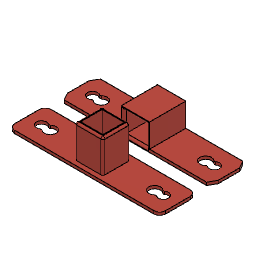
Solenoid v3 (Autodesk Fusion 360 design; units mm, degrees)
Autodesk Fusion 360 part; units mm, degrees
sketch "Sketch1" plane through (0, 0, 0) normal (0, 1, 0) x (1, 0, 0) in component "Solenoid base"
  line L0 (-25.5016, -20.45) -> (57.0484, -20.45)
  line L1 (57.0484, -20.45) -> (57.0484, -0.6062)
  line L2 (57.0484, -0.6062) -> (-25.5016, -0.6062)
  line L3 (-25.5016, -0.6062) -> (-25.5016, -20.45)
  dimension "d1_1_1" = 82.55
  dimension "d2_1_1" = 19.8438
  constraint horizontal L0
  constraint vertical L1
  constraint horizontal L2
  constraint vertical L3
  measures "d1_1_1" distance of L0.start L0.end
  measures "d2_1_1" distance of L0.end L1.end
extrude "Extrude1" add sketch "Sketch1" against normal blind 1.5875 makes body 1 in component "Solenoid base"
sketch "Sketch5" plane through (0, -1.5875, 0) normal (0, -1, 0) x (1, 0, 0) in component "Solenoid base"
  line L0 (15.7734, -11.3) -> (15.7734, 20.45) construction
  line L1 (46.9483, 10.5281) -> (-16.5517, 10.5281) construction
  line L2 (44.3484, 10.5281) -> (49.1109, 10.5281) construction
  arc A0 (47.5032, 8.2625) -> (46.5048, 8.1977) centre (47.0438, 7.6151) ccw
  arc A1 (46.5048, 12.8585) -> (47.5032, 12.7938) centre (47.0438, 13.4411) ccw
  arc A2 (47.5032, 8.2625) -> (47.5032, 12.7938) centre (49.1109, 10.5281) ccw
  arc A3 (46.5048, 12.8585) -> (46.5048, 8.1977) centre (44.3484, 10.5281) ccw
  arc A4 (-14.958, 8.1977) -> (-14.958, 12.8585) centre (-12.8016, 10.5281) ccw
  arc A5 (-15.9564, 12.7938) -> (-15.9564, 8.2625) centre (-17.5641, 10.5281) ccw
  arc A6 (-15.9564, 12.7938) -> (-14.958, 12.8585) centre (-15.497, 13.4411) ccw
  arc A7 (-14.958, 8.1977) -> (-15.9564, 8.2625) centre (-15.497, 7.6151) ccw
  line L3 (49.1109, 10.5281) -> (-12.8016, 10.5281) construction
  line L4 (57.0484, 10.5281) -> (-25.5016, 10.5281) construction
  line L5 (57.0484, 20.45) -> (-25.5016, 20.45)
  line L6 (-25.5016, 20.45) -> (-25.5016, 0.6062)
  line L7 (-25.5016, 0.6062) -> (57.0484, 0.6062)
  line L8 (57.0484, 0.6062) -> (57.0484, 20.45)
  dimension "d33_1_1" = 5.5563
  dimension "d35_1_1" = 1.5875
  dimension "d38_1_1" = 4.7625
  dimension "d40_1_1" = 3.175
  dimension "d2" = 28.575
  constraint coincident L2.end A2.centre
  constraint tangent A0 A2
  constraint horizontal L2
  constraint symmetric L2 A0.end A1.start
  constraint symmetric L2 A0.start A1.end
  constraint symmetric L2 A0 A1
  constraint tangent A0 A3
  constraint coincident L2.start A3.centre
  constraint symmetric L0 A0.end A4.start
  constraint symmetric L0 A0.start A5.end
  constraint symmetric L0 A0 A7
  constraint symmetric L0 A1.end A5.start
  constraint symmetric L0 A1.start A4.end
  constraint symmetric L0 A1 A6
  constraint symmetric L0 A2 A5
  constraint symmetric L0 A3 A4
  constraint coincident A4.centre L3.end
  constraint perpendicular L0 L3
  constraint collinear L1 L3
  constraint collinear L1 L4
  measures "d33_1_1" diameter of A2
  measures "d35_1_1" diameter of A0
  measures "d38_1_1" distance of L2.start L2.end
  measures "d40_1_1" radius of A3
  measures "d2" distance of L0 L2.start
extrude "Extrude12" cut sketch "Sketch5" against normal up to surface (1.5875 mm away) contours A0 A1 A2 A3 | A4 A5 A6 A7 bodies 1 in component "Solenoid base"
sketch "Sketch17" plane through (0, 0, 20.45) normal (0, 0, 1) x (1, 0, 0) in component "Solenoid base"
  line L0 (57.0484, 0) -> (-25.5016, 0)
  line L1 (-25.5016, -1.5875) -> (57.0484, -1.5875)
  line L2 (15.7734, 0) -> (15.7734, 14.8694) construction
  line L3 (15.7734, 0) -> (21.9329, 0)
  line L4 (21.9329, 0) -> (21.9329, 11.303)
  line L5 (21.9329, 11.303) -> (15.7734, 11.303)
  line L6 (9.6139, 0) -> (9.6139, 11.303)
  line L7 (9.6139, 11.303) -> (15.7734, 11.303)
  line L8 (8.0264, 0) -> (8.0264, 12.8905)
  line L9 (8.0264, 12.8905) -> (15.7734, 12.8905)
  line L10 (23.5204, 12.8905) -> (15.7734, 12.8905)
  line L11 (23.5204, -1.5875) -> (23.5204, 12.8905)
  line L12 (15.7734, -1.5875) -> (23.5204, -1.5875)
  line L13 (-25.5016, 0) -> (-25.5016, -1.5875)
  line L14 (57.0484, -1.5875) -> (57.0484, 0)
  dimension "d5" = 11.303
  dimension "d6" = 6.1595
  dimension "d7" = 1.5875
  constraint midpoint L0 L2.start
  constraint perpendicular L0 L2
  constraint horizontal L3
  constraint vertical L4
  constraint horizontal L5
  constraint symmetric L2 L3.end L6.start
  constraint symmetric L2 L4.end L6.end
  constraint symmetric L2 L5.end L7.end
  measures "d5" distance of L3 L5
  measures "d6" distance of L2 L4
extrude "Extrude13" add sketch "Sketch17" against normal up to surface (19.8438 mm away) contours L0 L4 L5 L6 L7 L8 L9 L10 L11 bodies 1 in component "Solenoid base"
sketch "Sketch1 (2)" plane through (0, 0, 0) normal (0, 1, 0) x (1, 0, 0) in component "Solenoid base vertical"
  line L0 (-25.5016, -20.45) -> (57.0484, -20.45)
  line L1 (57.0484, -20.45) -> (57.0484, -0.6062)
  line L2 (57.0484, -0.6062) -> (-25.5016, -0.6062)
  line L3 (-25.5016, -0.6062) -> (-25.5016, -20.45)
  dimension "d1_1_1_1" = 82.55
  dimension "d2_1_1_1" = 19.8438
  constraint horizontal L0
  constraint vertical L1
  constraint horizontal L2
  constraint vertical L3
  measures "d1_1_1_1" distance of L0.start L0.end
  measures "d2_1_1_1" distance of L0.end L1.end
extrude "Extrude1'" add sketch "Sketch1 (2)" against normal blind 1.5875 separate body makes body 2 in component "Solenoid base vertical"
sketch "Sketch5 (2)" plane through (0, -1.5875, 0) normal (0, -1, 0) x (1, 0, 0) in component "Solenoid base vertical"
  line L0 (15.7734, -11.3) -> (15.7734, 20.45) construction
  line L1 (46.9483, 10.5281) -> (-16.5517, 10.5281) construction
  line L2 (44.3484, 10.5281) -> (49.1109, 10.5281) construction
  arc A0 (47.5032, 8.2625) -> (46.5048, 8.1977) centre (47.0438, 7.6151) ccw
  arc A1 (46.5048, 12.8585) -> (47.5032, 12.7938) centre (47.0438, 13.4411) ccw
  arc A2 (47.5032, 8.2625) -> (47.5032, 12.7938) centre (49.1109, 10.5281) ccw
  arc A3 (46.5048, 12.8585) -> (46.5048, 8.1977) centre (44.3484, 10.5281) ccw
  arc A4 (-14.958, 8.1977) -> (-14.958, 12.8585) centre (-12.8016, 10.5281) ccw
  arc A5 (-15.9564, 12.7938) -> (-15.9564, 8.2625) centre (-17.5641, 10.5281) ccw
  arc A6 (-15.9564, 12.7938) -> (-14.958, 12.8585) centre (-15.497, 13.4411) ccw
  arc A7 (-14.958, 8.1977) -> (-15.9564, 8.2625) centre (-15.497, 7.6151) ccw
  line L3 (49.1109, 10.5281) -> (-12.8016, 10.5281) construction
  line L4 (57.0484, 10.5281) -> (-25.5016, 10.5281) construction
  line L5 (57.0484, 20.45) -> (-25.5016, 20.45)
  line L6 (-25.5016, 20.45) -> (-25.5016, 0.6062)
  line L7 (-25.5016, 0.6062) -> (57.0484, 0.6062)
  line L8 (57.0484, 0.6062) -> (57.0484, 20.45)
  dimension "d33_1_1_1" = 5.5563
  dimension "d35_1_1_1" = 1.5875
  dimension "d38_1_1_1" = 4.7625
  dimension "d40_1_1_1" = 3.175
  dimension "d2_2" = 28.575
  constraint coincident L2.end A2.centre
  constraint tangent A0 A2
  constraint horizontal L2
  constraint symmetric L2 A0.end A1.start
  constraint symmetric L2 A0.start A1.end
  constraint symmetric L2 A0 A1
  constraint tangent A0 A3
  constraint coincident L2.start A3.centre
  constraint symmetric L0 A0.end A4.start
  constraint symmetric L0 A0.start A5.end
  constraint symmetric L0 A0 A7
  constraint symmetric L0 A1.end A5.start
  constraint symmetric L0 A1.start A4.end
  constraint symmetric L0 A1 A6
  constraint symmetric L0 A2 A5
  constraint symmetric L0 A3 A4
  constraint coincident A4.centre L3.end
  constraint perpendicular L0 L3
  constraint collinear L1 L3
  constraint collinear L1 L4
  measures "d33_1_1_1" diameter of A2
  measures "d35_1_1_1" diameter of A0
  measures "d38_1_1_1" distance of L2.start L2.end
  measures "d40_1_1_1" radius of A3
  measures "d2_2" distance of L0 L2.start
extrude "Extrude12'" cut sketch "Sketch5 (2)" against normal up to surface (1.5875 mm away) contours A0 A1 A2 A3 | A4 A5 A6 A7 bodies 2 in component "Solenoid base vertical"
sketch "Sketch17 (2)" plane through (0, 0, 20.45) normal (0, 0, 1) x (1, 0, 0) in component "Solenoid base vertical"
  line L0 (57.0484, 0) -> (-25.5016, 0)
  line L1 (-25.5016, -1.5875) -> (57.0484, -1.5875)
  line L2 (15.7734, 0) -> (15.7734, 14.8694) construction
  line L3 (15.7734, 0) -> (22.9172, 0)
  line L4 (22.9172, 0) -> (22.9172, 14.2875)
  line L5 (22.9172, 14.2875) -> (15.7734, 14.2875)
  line L6 (8.6297, 0) -> (8.6297, 14.2875)
  line L7 (8.6297, 14.2875) -> (15.7734, 14.2875)
  line L8 (7.0422, 0) -> (7.0422, 15.875)
  line L9 (7.0422, 15.875) -> (15.7734, 15.875)
  line L10 (24.5047, 15.875) -> (15.7734, 15.875)
  line L11 (24.5047, -1.5875) -> (24.5047, 15.875)
  line L12 (15.7734, -1.5875) -> (24.5047, -1.5875)
  line L13 (-25.5016, 0) -> (-25.5016, -1.5875)
  line L14 (57.0484, -1.5875) -> (57.0484, 0)
  dimension "d5_2" = 14.2875
  dimension "d6_2" = 7.1437
  dimension "d7_2" = 1.5875
  constraint midpoint L0 L2.start
  constraint perpendicular L0 L2
  constraint horizontal L3
  constraint vertical L4
  constraint horizontal L5
  constraint symmetric L2 L3.end L6.start
  constraint symmetric L2 L4.end L6.end
  constraint symmetric L2 L5.end L7.end
  measures "d5_2" distance of L3 L5
  measures "d6_2" distance of L2 L4
sketch "Sketch18" plane through (0, 0, 0) normal (0, 1, 0) x (-1, 0, 0) in component "Solenoid base vertical"
  arc A0 (-46.5048, 8.1977) -> (-47.5032, 8.2625) centre (-47.0438, 7.6151) ccw
  arc A1 (-47.5032, 12.7938) -> (-47.5032, 8.2625) centre (-49.1109, 10.5281) ccw
  arc A2 (-47.5032, 12.7938) -> (-46.5048, 12.8585) centre (-47.0438, 13.4411) ccw
  arc A3 (-46.5048, 8.1977) -> (-46.5048, 12.8585) centre (-44.3484, 10.5281) ccw
  arc A4 (14.958, 12.8585) -> (15.9564, 12.7938) centre (15.497, 13.4411) ccw
  arc A5 (15.9564, 8.2625) -> (15.9564, 12.7938) centre (17.5641, 10.5281) ccw
  arc A6 (15.9564, 8.2625) -> (14.958, 8.1977) centre (15.497, 7.6151) ccw
  arc A7 (14.958, 12.8585) -> (14.958, 8.1977) centre (12.8016, 10.5281) ccw
  line L0 (25.5016, 0.6062) -> (25.5016, 20.45)
  line L1 (25.5016, 20.45) -> (-57.0484, 20.45)
  line L2 (-57.0484, 20.45) -> (-57.0484, 0.6062)
  line L3 (-57.0484, 0.6062) -> (25.5016, 0.6062)
  line L4 (-15.7734, 0.6062) -> (-15.7734, 20.45) construction
  line L5 (-8.6297, 0.6062) -> (-22.9172, 0.6062)
  line L6 (-21.8694, 4.6861) -> (-21.8694, 16.3701)
  line L7 (-22.9172, 20.45) -> (-8.6297, 20.45)
  line L8 (-9.6774, 16.3701) -> (-9.6774, 4.6861)
  line L9 (-9.6774, 4.6861) -> (-21.8694, 4.6861)
  line L10 (-21.8694, 10.5281) -> (-21.8694, 16.3701)
  line L11 (-21.8694, 16.3701) -> (-9.6774, 16.3701)
  line L12 (-9.6774, 10.5281) -> (-9.6774, 4.6861)
  line L13 (-9.6774, 10.5281) -> (-27.6863, 10.5281) construction
  line L14 (25.5016, 10.5281) -> (-3.8857, 10.5281) construction
  dimension "d10" = 6.096
  dimension "d11" = 12.192
  dimension "d12" = 11.684
  dimension "d14" = 5.842
  constraint midpoint L3 L4.start
  constraint midpoint L1 L4.end
  constraint horizontal L5
  constraint vertical L6
  constraint horizontal L7
  constraint vertical L8
  constraint coincident L1 L7.start
  constraint coincident L3 L5.start
  constraint horizontal L9
  constraint vertical L10
  constraint horizontal L11
  constraint vertical L12
  constraint perpendicular L6 L13
  constraint coincident L8 L12.start
  constraint midpoint L0 L14.start
  constraint perpendicular L0 L14
  constraint coincident L13 L10.start
  measures "d10" distance of L4 L6
  measures "d11" distance of L6 L8
  measures "d12" distance of L6.start L6.end
  measures "d14" distance of L9 L14
extrude "Extrude14" cut sketch "Sketch18" against normal up to surface (1.5875 mm away) contours L6 L8 L9 L10 L11 L12 bodies 2 in component "Solenoid base vertical"
sketch "Sketch19" plane through (0, 0, 0) normal (0, 1, 0) x (-1, 0, 0) in component "Solenoid base vertical"
  line L0 (-9.6774, 4.6861) -> (-21.8694, 4.6861)
  line L1 (-21.8694, 4.6861) -> (-21.8694, 16.3701)
  line L2 (-21.8694, 16.3701) -> (-9.6774, 16.3701)
  line L3 (-9.6774, 16.3701) -> (-9.6774, 4.6861)
  arc A0 (-46.5048, 8.1977) -> (-47.5032, 8.2625) centre (-47.0438, 7.6151) ccw
  arc A1 (-47.5032, 12.7938) -> (-47.5032, 8.2625) centre (-49.1109, 10.5281) ccw
  arc A2 (-47.5032, 12.7938) -> (-46.5048, 12.8585) centre (-47.0438, 13.4411) ccw
  arc A3 (-46.5048, 8.1977) -> (-46.5048, 12.8585) centre (-44.3484, 10.5281) ccw
  arc A4 (14.958, 12.8585) -> (15.9564, 12.7938) centre (15.497, 13.4411) ccw
  arc A5 (15.9564, 8.2625) -> (15.9564, 12.7938) centre (17.5641, 10.5281) ccw
  arc A6 (15.9564, 8.2625) -> (14.958, 8.1977) centre (15.497, 7.6151) ccw
  arc A7 (14.958, 12.8585) -> (14.958, 8.1977) centre (12.8016, 10.5281) ccw
  line L4 (25.5016, 0.6062) -> (25.5016, 20.45)
  line L5 (25.5016, 20.45) -> (-57.0484, 20.45)
  line L6 (-57.0484, 20.45) -> (-57.0484, 0.6062)
  line L7 (-57.0484, 0.6062) -> (25.5016, 0.6062)
  line L8 (-23.4569, 17.9576) -> (-8.0899, 17.9576)
  line L9 (-8.0899, 17.9576) -> (-8.0899, 3.0986)
  line L10 (-8.0899, 3.0986) -> (-23.4569, 3.0986)
  line L11 (-23.4569, 3.0986) -> (-23.4569, 17.9576)
  dimension "d17" = -1.5875
extrude "Extrude15" add sketch "Sketch19" along normal blind 18.0086 contours L8 L9 L10 L11 bodies 2 in component "Solenoid base vertical"
fillet "Fillet9" radius 1.0922 8 edges at (23.4569, 9.0043, 17.9576) (23.4569, 9.0043, 3.0986) (8.0899, 9.0043, 3.0986) (8.0899, 9.0043, 17.9576) (8.0899, 18.0086, 10.5281) (15.7734, 18.0086, 17.9576) (23.4569, 18.0086, 10.5281) (15.7734, 18.0086, 3.0986) on bodies 2 in component "Solenoid base vertical"
fillet "Fillet10" radius 3.175 4 edges at (57.0484, -0.7937, 20.45) (57.0484, -0.7937, 0.6062) (-25.5016, -0.7937, 20.45) (-25.5016, -0.7937, 0.6062) on bodies 2 in component "Solenoid base vertical"
fillet "Fillet9'" radius 1.27 4 edges at (15.7734, 0, 20.45) (9.6139, 5.6515, 20.45) (15.7734, 11.303, 20.45) (21.9329, 5.6515, 20.45) on bodies 1 in component "Solenoid base"
sketch "Sketch18 (2)" plane through (0, -1.5875, 0) normal (0, -1, 0) x (1, 0, 0) in component "Solenoid base"
  arc A0 (47.5032, 8.2625) -> (46.5048, 8.1977) centre (47.0438, 7.6151) ccw
  arc A1 (46.5048, 12.8585) -> (46.5048, 8.1977) centre (44.3484, 10.5281) ccw
  arc A2 (46.5048, 12.8585) -> (47.5032, 12.7938) centre (47.0438, 13.4411) ccw
  arc A3 (47.5032, 8.2625) -> (47.5032, 12.7938) centre (49.1109, 10.5281) ccw
  arc A4 (-15.9564, 12.7938) -> (-14.958, 12.8585) centre (-15.497, 13.4411) ccw
  arc A5 (-14.958, 8.1977) -> (-14.958, 12.8585) centre (-12.8016, 10.5281) ccw
  arc A6 (-14.958, 8.1977) -> (-15.9564, 8.2625) centre (-15.497, 7.6151) ccw
  arc A7 (-15.9564, 12.7938) -> (-15.9564, 8.2625) centre (-17.5641, 10.5281) ccw
  line L0 (-25.5016, 20.45) -> (-25.5016, 0.6062)
  line L1 (-25.5016, 0.6062) -> (57.0484, 0.6062)
  line L2 (57.0484, 0.6062) -> (57.0484, 20.45)
  line L3 (57.0484, 20.45) -> (-25.5016, 20.45)
  line L4 (-23.2102, 20.45) -> (-25.5016, 16.4812)
  line L5 (-23.2102, 20.45) -> (-25.5016, 20.45)
  line L6 (-25.5016, 16.4812) -> (-25.5016, 20.45)
  line L7 (15.7734, 20.45) -> (15.7734, 4.7728) construction
  line L8 (8.0264, 20.45, -1.5875) -> (8.0264, 0.6062, -1.5875)
  line L9 (54.757, 20.45) -> (57.0484, 20.45)
  line L10 (54.757, 20.45) -> (57.0484, 16.4812)
  line L11 (57.0484, 16.4812) -> (57.0484, 20.45)
  line L12 (57.0484, 10.5281) -> (23.201, 10.5281) construction
  line L13 (54.757, 0.6062) -> (57.0484, 4.575)
  line L14 (57.0484, 4.575) -> (57.0484, 0.6062)
  line L15 (54.757, 0.6062) -> (57.0484, 0.6062)
  line L16 (-23.2102, 0.6062) -> (-25.5016, 4.575)
  line L17 (-23.2102, 0.6062) -> (-25.5016, 0.6062)
  line L18 (-25.5016, 4.575) -> (-25.5016, 0.6062)
  point P0 (57.0484, 20.45)
  dimension "d23" = 30
  dimension "d24" = 3.9688
  constraint coincident L3 L4.start
  constraint coincident L0 L4.end
  constraint coincident L0.start L3.end
  constraint midpoint L3 L7.start
  constraint perpendicular L3 L7
  constraint symmetric L0.start L7 P0
  constraint symmetric L4.start L7 L9.start
  constraint symmetric L4.end L7 L10.end
  constraint midpoint L2 L12.start
  constraint perpendicular L2 L12
  constraint symmetric L4.start L12 L16.start
  constraint symmetric L4.end L12 L16.end
  constraint symmetric L0.start L12 L0.end
  constraint symmetric L9.start L12 L13.start
  constraint symmetric P0 L12 L1.end
  constraint symmetric L10.end L12 L13.end
  measures "d23" angle of L0 L4
  measures "d24" distance of L0.start L4.end
extrude "Extrude14'" cut sketch "Sketch18 (2)" against normal up to surface (1.5875 mm away) contours L0 L3 L4 L5 L6 | L0 L1 L16 L17 L18 | L2 L3 L9 L10 L11 | L1 L2 L13 L14 L15 bodies 1 in component "Solenoid base"
component "Solenoid base" placed x (1, 0, 0) y (0, 1, 0) z (0, 0, 1) at (0, 0, 0)
component "Solenoid base vertical" placed x (1, 0, 0) y (0, 1, 0) z (0, 0, 1) at (0, 0, 27.94)
equation "d3_1_1 = d1_1_1 / 2 - 0.246 in"
equation "d4_1_1 = ( d2_1_1 - 0.889764 in ) / 2"
equation "d8_1_1 = 0.25 in"
equation "d10_1_1 = 2.50 in / 2"
equation "d14_1_1 = 0.889764 in / 2 + d16_1_1 / 2"
equation "d16_1_1 = 0.25 in"
equation "d30_1_1 = 0.063 in"
equation "d33_1_1 = 0.25 in - 0.03125 in"
equation "d36_1_1 = ( 1.25 in ) / 2 - d32_1"
equation "d41_1_1 = -0.40 in"
equation "d42_1_1 = 0.0 deg"
equation "d65_1 = 0.89 in"
equation "d66_1 = d65_1"
equation "d67_1 = 0.00 in"
equation "d75_1 = 0.09375 in"
equation "d78_1 = d75_1"
equation "d93_1 = 0.625 in + d75_1 / 2"
equation "d95_1 = 0.1875 in + 0.010 in"
equation "d96_1 = 0.0 deg"
equation "d97_1 = 0.0625 in"
equation "d98_1 = 0.0 deg"
equation "d99_1 = 0.8900 in"
equation "d100_1 = 0.1875 in + 0.01 in"
equation "d101_1 = 0.0 deg"
equation "d102_1 = 0.06250 in"
equation "d103_1 = 0.0 deg"
equation "d104_1 = -0.3125 in"
equation "d105_1 = -10.0 deg"
equation "d106_1 = -0.25 in"
equation "d107_1 = 0.0 deg"
equation "d108_1 = 0.09375 in"
equation "d109_1 = d108_1"
equation "d110_1 = -0.2500 in"
equation "d111_1 = 0.0 deg"
equation "d115_1 = 0.060 in"
equation "d116_1 = 0.030 in"
equation "d117_1 = 0.25 in"
equation "d118_1 = 90.0 deg"
equation "d119_1 = 90.0 deg"
equation "d32_1 = 0.25 in + ( 0.03125 / 2 ) * 1 in"
equation "d6 = ( 0.485 / 2 ) * 1 in"
equation "d33_1_1_1 = 0.25 in - 0.03125 in"
equation "d6_2 = ( 0.5625 / 2 ) * 1 in"
equation "d10 = d11 / 2"
equation "d14 = d12 / 2"
